Autodesk Fusion 360 part; units mm, degrees
(part 2 of 2)
extrude "押し出し20" add sketch "スケッチ19" against normal blind 3.5 separate body contours A4 makes body 4
extrude "押し出し21" add sketch "スケッチ19" along normal blind 6.5 contours L1 L2 L10 L11 L16 L17 L18 L19 A2 A5 | L1 L2 L3 A2 A5 | L11 A2 | L2 L3 L9 L10 L14 L15 L16 L19 A2 A5 | L9 A2 | L2 L16 L24 L25 | L2 A5 L24 L25 | L16 L17 A5 | L10 A2 A5 | L16 A3 L24 L25 | L15 L16 A5 | A3 | L17 A5 L26 L27 | L17 A3 L26 L27 | L10 A5 L20 L21 | L10 L19 L20 L21 | L17 L18 L19 A5 | L19 A3 L20 L21 | L14 L15 L19 A5 | L15 A3 L22 L23 | L15 A5 L22 L23 | A4 bodies 4
extrude "押し出し22" cut 1 faces at (24.2955, 69.1575, -2.5) along direction (0, 0, -1) blind 1 on bodies 4 bodies 4
sketch "スケッチ20" plane through (0, 0, -9) normal (0, 0, -1) x (-1, 0, 0)
  circle A0 centre (0, 67.4909) radius 2
  line L0 (32.1131, 72.4909) -> (8.6603, 72.4909)
  arc A1 (8.6603, 72.4909) -> (5, 76.1511) centre (0, 67.4909) ccw
  line L1 (5, 76.1511) -> (5, 99.604)
  arc A2 (32.1131, 72.4909) -> (5, 99.604) centre (0, 67.4909) ccw
  arc A3 (-5, 99.604) -> (-32.1131, 72.4909) centre (0, 67.4909) ccw
  line L2 (-5, 99.604) -> (-5, 76.1511)
  arc A4 (-5, 76.1511) -> (-8.6603, 72.4909) centre (0, 67.4909) ccw
  line L3 (-8.6603, 72.4909) -> (-32.1131, 72.4909)
  arc A5 (5, 58.8306) -> (8.6603, 62.4909) centre (0, 67.4909) ccw
  line L4 (8.6603, 62.4909) -> (32.1131, 62.4909)
  arc A6 (5, 35.3778) -> (32.1131, 62.4909) centre (0, 67.4909) ccw
  line L5 (5, 35.3778) -> (5, 58.8306)
  arc A7 (-8.6603, 62.4909) -> (-5, 58.8306) centre (0, 67.4909) ccw
  line L6 (-5, 58.8306) -> (-5, 35.3778)
  arc A8 (-32.1131, 62.4909) -> (-5, 35.3778) centre (0, 67.4909) ccw
  line L7 (-32.1131, 62.4909) -> (-8.6603, 62.4909)
  circle A9 centre (0, 67.4909) radius 40
  circle A10 centre (0, 67.4909) radius 2
  dimension "d120" = 4
  constraint concentric A0 A10
  measures "d120" diameter of A10
extrude "押し出し23" add sketch "スケッチ20" against normal blind 0.9 contours A0 A10 bodies 4
sketch "スケッチ21" plane through (0, 0, 22.5) normal (0, 0, 1) x (1, 0, 0)
  circle A0 centre (12.5, 67.4909) radius 1.5
  circle A1 centre (0, 57.9909) radius 1.5
  circle A2 centre (-33.6231, 90.7231) radius 1.5
  circle A3 centre (0, 67.4909) radius 4
  circle A4 centre (31.8909, 38.8909) radius 1.5
  circle A5 centre (-31.8909, 38.8909) radius 1.5
  circle A6 centre (-12.5, 67.4909) radius 1.5
  circle A7 centre (33.6231, 90.7231) radius 1.5
  circle A8 centre (0, 76.9909) radius 1.5
  line L0 (-25, 88.9909) -> (-25, 95.9909)
  line L1 (-25, 95.9909) -> (-38.8909, 95.9909)
  line L2 (-38.8909, 95.9909) -> (-38.8909, 38.8909)
  line L3 (-38.8909, 38.8909) -> (-31.6632, 31.6632)
  line L4 (-31.6632, 31.6632) -> (31.6632, 31.6632)
  line L5 (31.6632, 31.6632) -> (38.8909, 38.8909)
  line L6 (38.8909, 38.8909) -> (38.8909, 95.9909)
  line L7 (38.8909, 95.9909) -> (25, 95.9909)
  line L8 (25, 95.9909) -> (25, 88.9909)
  line L9 (25, 88.9909) -> (-25, 88.9909)
  circle A9 centre (0, 76.9909) radius 3.25
  circle A10 centre (12.5, 67.4909) radius 3.25
  circle A11 centre (-12.5, 67.4909) radius 3.25
  circle A12 centre (0, 57.9909) radius 3.25
  dimension "d123" = 6.5
  dimension "d124" = 6.5
  dimension "d125" = 6.5
  dimension "d126" = 6.5
  constraint concentric A8 A9
  constraint concentric A0 A10
  constraint concentric A6 A11
  constraint concentric A1 A12
  measures "d123" diameter of A9
  measures "d124" diameter of A10
  measures "d125" diameter of A11
  measures "d126" diameter of A12
extrude "押し出し24" cut sketch "スケッチ21" against normal blind 3 contours A9 | A10 | A11 | A12 bodies 2
ref_plane "作業平面1" through (0, 63.827, 26) normal (0, 0, 1) x (1, 0, 0)
sketch "スケッチ22" plane through (0, 0, 26) normal (0, 0, 1) x (1, 0, 0)
  circle A0 centre (0, 67.4909) radius 3.25
  line L0 (10.7, 57.3309) -> (-10.7, 57.3309)
  line L1 (-12.7, 59.3309) -> (-12.7, 75.6509)
  line L2 (-10.7, 77.6509) -> (10.7, 77.6509)
  line L3 (12.7, 75.6509) -> (12.7, 59.3309)
  line L4 (12.7, 57.3309) -> (-12.7, 77.6509) construction
  line L5 (-12.7, 57.3309) -> (12.7, 77.6509) construction
  circle A1 centre (-10.1, 75.0509) radius 1.1
  circle A2 centre (10.1, 75.0509) radius 1.1
  circle A3 centre (-10.1, 59.9309) radius 1.1
  circle A4 centre (10.1, 59.9309) radius 1.1
  arc A5 (-10.7, 77.6509) -> (-12.7, 75.6509) centre (-10.7, 75.6509) ccw
  arc A6 (12.7, 75.6509) -> (10.7, 77.6509) centre (10.7, 75.6509) ccw
  arc A7 (10.7, 57.3309) -> (12.7, 59.3309) centre (10.7, 59.3309) ccw
  arc A8 (-12.7, 59.3309) -> (-10.7, 57.3309) centre (-10.7, 59.3309) ccw
  point P0 (0, 67.4909)
  dimension "d130" = 20.32
  dimension "d131" = 25.4
  dimension "d132" = 2.2
  dimension "d133" = 2.2
  dimension "d134" = 2.2
  dimension "d135" = 2.2
  dimension "d136" = 2.6
  dimension "d137" = 2.6
  dimension "d138" = 2.6
  dimension "d139" = 2.6
  dimension "d140" = 2.6
  dimension "d141" = 2.6
  dimension "d142" = 2.6
  dimension "d143" = 2.6
  dimension "d144" = 2
  constraint horizontal L0
  constraint perpendicular L0 L1
  constraint parallel L0 L2
  constraint parallel L1 L3
  constraint coincident L4 P0
  constraint coincident L5 P0
  constraint coincident P0 A0.centre
  constraint coincident L4.end L2
  constraint coincident L4.end L1
  constraint tangent L2 A5
  constraint tangent L1 A5
  constraint coincident L5.end L2
  constraint coincident L5.end L3
  constraint tangent L2 A6
  constraint tangent L3 A6
  constraint equal A5 A6
  constraint coincident L4.start L0
  constraint coincident L4.start L3
  constraint tangent L0 A7
  constraint tangent L3 A7
  constraint equal A5 A7
  constraint coincident L5.start L1
  constraint coincident L5.start L0
  constraint tangent L1 A8
  constraint tangent L0 A8
  constraint equal A5 A8
  measures "d130" distance of L5.start L4.end
  measures "d131" distance of L4.end L5.end
  measures "d132" diameter of A1
  measures "d133" diameter of A2
  measures "d134" diameter of A3
  measures "d135" diameter of A4
  measures "d136" distance of L3 A4.centre
  measures "d137" distance of L1 A3.centre
  measures "d138" distance of L3 A2.centre
  measures "d139" distance of L1 A1.centre
  measures "d140" distance of L2 A1.centre
  measures "d141" distance of L2 A2.centre
  measures "d142" distance of L0 A4.centre
  measures "d143" distance of L0 A3.centre
  measures "d144" radius of A5
extrude "押し出し25" add sketch "スケッチ22" along normal blind 1.5 separate body contours A0 | L0 L1 L2 L3 A5 A6 A7 A8 makes body 5
sketch "スケッチ23" plane through (0, 0, 26) normal (0, 0, -1) x (-1, 0, 0)
  circle A0 centre (10.1, 59.9309) radius 1.1
  circle A1 centre (-10.1, 75.0509) radius 1.1
  circle A2 centre (-10.1, 59.9309) radius 1.1
  circle A3 centre (10.1, 75.0509) radius 1.1
  arc A4 (12.7, 75.6509) -> (10.7, 77.6509) centre (10.7, 75.6509) ccw
  line L0 (10.7, 77.6509) -> (-10.7, 77.6509)
  arc A5 (-10.7, 77.6509) -> (-12.7, 75.6509) centre (-10.7, 75.6509) ccw
  line L1 (-12.7, 75.6509) -> (-12.7, 59.3309)
  arc A6 (-12.7, 59.3309) -> (-10.7, 57.3309) centre (-10.7, 59.3309) ccw
  line L2 (-10.7, 57.3309) -> (10.7, 57.3309)
  arc A7 (10.7, 57.3309) -> (12.7, 59.3309) centre (10.7, 59.3309) ccw
  line L3 (12.7, 59.3309) -> (12.7, 75.6509)
  line L4 (-8.1, 75.0509) -> (-8.1, 78.0509)
  line L5 (-8.1, 78.0509) -> (-13.1, 78.0509)
  line L6 (-13.1, 78.0509) -> (-13.1, 73.0509)
  line L7 (-13.1, 73.0509) -> (-10.1, 73.0509)
  arc A8 (-10.1, 73.0509) -> (-8.1, 75.0509) centre (-10.1, 75.0509) ccw
  line L8 (-10.1, 61.9309) -> (-13.1, 61.9309)
  line L9 (-13.1, 61.9309) -> (-13.1, 56.9309)
  line L10 (-13.1, 56.9309) -> (-8.1, 56.9309)
  line L11 (-8.1, 56.9309) -> (-8.1, 59.9309)
  line L12 (8.1, 75.0509) -> (8.1, 78.0509)
  line L13 (8.1, 78.0509) -> (13.1, 78.0509)
  line L14 (13.1, 78.0509) -> (13.1, 73.0509)
  line L15 (13.1, 73.0509) -> (10.1, 73.0509)
  line L16 (10.1, 61.9309) -> (13.1, 61.9309)
  line L17 (13.1, 61.9309) -> (13.1, 56.9309)
  line L18 (13.1, 56.9309) -> (8.1, 56.9309)
  line L19 (8.1, 56.9309) -> (8.1, 59.9309)
  arc A9 (8.1, 75.0509) -> (10.1, 73.0509) centre (10.1, 75.0509) ccw
  arc A10 (10.1, 61.9309) -> (8.1, 59.9309) centre (10.1, 59.9309) ccw
  arc A11 (-8.1, 59.9309) -> (-10.1, 61.9309) centre (-10.1, 59.9309) ccw
  circle A12 centre (-10.1, 75.0509) radius 1.05
  circle A13 centre (10.1, 75.0509) radius 1.05
  circle A14 centre (10.1, 59.9309) radius 1.05
  circle A15 centre (-10.1, 59.9309) radius 1.05
  dimension "d147" = 4
  dimension "d149" = 4
  dimension "d150" = 4
  dimension "d151" = 4
  dimension "d152" = 3
  dimension "d153" = 3
  dimension "d154" = 3
  dimension "d155" = 3
  dimension "d156" = 3
  dimension "d157" = 3
  dimension "d159" = 3
  dimension "d160" = 3
  dimension "d161" = 2.1
  dimension "d162" = 2.1
  dimension "d163" = 2.1
  dimension "d164" = 2.1
  constraint concentric A3 A9
  constraint concentric A0 A10
  constraint concentric A1 A8
  constraint concentric A2 A11
  constraint tangent L7 A8
  constraint tangent L4 A8
  constraint vertical L6
  constraint horizontal L7
  constraint vertical L4
  constraint horizontal L5
  constraint tangent L11 A11
  constraint tangent L8 A11
  constraint horizontal L8
  constraint vertical L11
  constraint horizontal L10
  constraint vertical L9
  constraint tangent L15 A9
  constraint tangent L16 A10
  constraint tangent L19 A10
  constraint tangent L12 A9
  constraint horizontal L15
  constraint vertical L12
  constraint horizontal L13
  constraint vertical L14
  constraint horizontal L16
  constraint vertical L19
  constraint horizontal L18
  constraint vertical L17
  constraint concentric A8 A12
  constraint concentric A9 A13
  constraint concentric A10 A14
  constraint concentric A11 A15
  measures "d147" diameter of A9
  measures "d149" diameter of A10
  measures "d150" diameter of A8
  measures "d151" diameter of A11
  measures "d152" distance of L4.start L4.end
  measures "d153" distance of L6.end L7.end
  measures "d154" horizontal distance of L8.start L8.end
  measures "d155" distance of L10.end L11.end
  measures "d156" distance of L16.start L16.end
  measures "d157" distance of L18.end L19.end
  measures "d159" distance of L14.end L15.end
  measures "d160" distance of L12.start L12.end
  measures "d161" diameter of A12
  measures "d162" diameter of A13
  measures "d163" diameter of A14
  measures "d164" diameter of A15
extrude "押し出し26" add sketch "スケッチ23" along normal blind 3.5 contours A4 L0 L3 L12 L15 A9 | A4 L0 L3 L12 L13 L14 L15 | L2 A7 L3 L16 L17 L18 L19 | L2 A7 L3 L16 L19 A10 | L0 A5 L1 L4 L7 A8 | L0 A5 L1 L4 L5 L6 L7 | L1 A6 L2 L8 L9 L10 L11 | L1 A6 L2 L8 L11 A11 bodies 2
extrude "押し出し27" cut 4 faces at (-10.679, 59.6107, 22.5) (-9.668, 75.3003, 22.5) (9.541, 75.3364, 22.5) (10.532, 60.1803, 22.5) along direction (0, 0, -1) blind 1 on bodies 2 bodies 2
named bodies: "モータ取り付け台", "BLDC", "リアクションホイール", "磁気エンコーダ"
